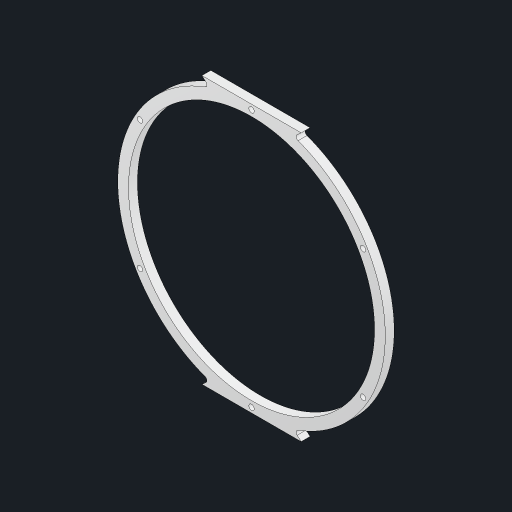
# Autodesk Inventor part: Weapon Disk
Saved by Autodesk Inventor 2023.2 (Build 272271030, 271C)
## iProperties
Created: 2024-02-21
Part Number: Weapon Disk
Material: Aluminum 6061
Document SubType Name: Modeling
Designer: robpl
Density: 2.7 g/cm^3
Appearance: Aluminum - Flat
Mass: 33.3647 g
Surface Area: 99.8313 cm^2
Volume: 12.3573 cm^3
Author: robpl
Autodesk Inventor part; units mm, degrees
ref_plane "YZ Plane" through (0, 0, 0) normal (1, 0, 0) x (0, 1, 0)
ref_plane "XZ Plane" through (0, 0, 0) normal (0, 1, 0) x (-1, 0, 0)
ref_plane "XY Plane" through (0, 0, 0) normal (0, 0, 1) x (1, 0, 0)
sketch "Sketch1" plane through (0, 0, 0) normal (0, 0, 1) x (1, 0, 0)
  circle A0 centre (0, 0) radius 69
  circle A1 centre (0, 0) radius 75
  line L0 (0, 75) -> (27.8388, 75)
  line L1 (27.8388, 75) -> (0, 0)
  line L2 (27.8388, 75) -> (23.5579, 71.2041)
  arc A2 (25.5942, 73.0097) -> (26.0989, 70.3125) centre (26.6557, 71.8125) ccw
  line L3 (0, 0) -> (23.5794, 0)
  line L4 (0, -75) -> (-27.8388, -75)
  line L5 (-27.8388, -75) -> (-23.5579, -71.2041)
  arc A3 (-25.5942, -73.0097) -> (-26.0989, -70.3125) centre (-26.6557, -71.8125) ccw
  line L6 (0, 0) -> (0, 17.5372)
  point P0 (-26.0989, -70.3125)
  dimension "d0" = 138
  dimension "d1" = 150
  dimension "d2" = 5
  dimension "d3" = 1.6
  dimension "d6" = 360
  constraints: 14 end point, 7 point on circle, 4 centre point, 3 point on line, 2 coincident, 2 horizontal, 2 tangent, 1 vertical, 1 vertical alignment, 19 other
  measures "d0" diameter of A0
  measures "d1" diameter of A1
  measures "d2" distance of L0.end A2.end
  measures "d3" radius of A2
extrude "Extrusion1" add sketch "Sketch1" along normal blind 5 contours A1
extrude "Extrusion2" add sketch "Sketch1" along normal blind 5 contours A1 L2 A2 | A1 L0 L2
mirror "Mirror1" about plane through (0, 0, 0) normal (0, 1, 0) of "Extrusion2"
mirror "Mirror2" about plane through (0, 0, 0) normal (1, 0, 0) of "Extrusion2", "Mirror1"
sketch "Sketch2" plane through (0, 0, 5) normal (0, 0, 1) x (1, 0, 0)
  circle A0 centre (0, 72.25) radius 1.5
  arc A1 (26.0989, -70.3125) -> (26.0989, 70.3125) centre (0, 0) ccw projected
  circle A2 centre (0, 0) radius 75
  circle A3 centre (0, 72.25) radius 2.75
  point P0 (0, 69.5)
  dimension "d23" = 5.5
  dimension "d12" = 3
  constraints: 3 vertical alignment, 2 coincident, 1 centre point, 5 other
  measures "d12" diameter of A0
extrude "Extrusion3" cut sketch "Sketch2" against normal blind 5 contours A0
sketch "Sketch3" plane through (0, 0, 5) normal (0, 0, 1) x (1, 0, 0)
  circle A0 centre (0, 72.25) radius 1.5 projected
  circle A1 centre (0, 72.25) radius 2.75
  line L0 (-27.8388, 75) -> (27.8388, 75) projected
  circle A2 centre (0, 72.25) radius 2.4563
  point P0 (0, 0)
  point P1 (-0.97, 69.9933)
  point P2 (0.97, 69.9933)
  point P3 (-0.97, 69.9933)
  constraints: 2 coincident, 1 centre point, 1 tangent, 4 other
extrude "Extrusion4" [suppressed]
fillet "Fillet1" [suppressed]
pattern_circular "Circular Pattern1" count 6 over 360 about axis through (0, 0, 0) along (0, 0, 1) of "Extrusion3"
body "Solid1"
